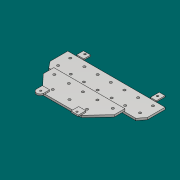
# Autodesk Inventor part: plastic_mount
Saved by Autodesk Inventor 2018 (Build 220112000, 112)
## iProperties
Created: 2021-07-30
Part Number: plastic_mount
Material: アルミニウム 6061
Document SubType Name: Modeling
Designer: gisen
Density: 2.7 g/cm^3
Appearance: アルミニウム - フラット
Author: gisen
Autodesk Inventor part; units mm, degrees
ref_plane "YZ Plane" through (0, 0, 0) normal (1, 0, 0) x (0, 1, 0)
ref_plane "XZ Plane" through (0, 0, 0) normal (0, 1, 0) x (-1, 0, 0)
ref_plane "XY Plane" through (0, 0, 0) normal (0, 0, 1) x (1, 0, 0)
sketch "スケッチ1" plane through (0, 0, 0) normal (0, 0, 1) x (1, 0, 0)
  line L0 (-67.1, 0) -> (-67.1, -24.4741)
  line L1 (-67.1, -24.4741) -> (-60, -33.4)
  line L2 (-60, -33.4) -> (60, -33.4)
  line L3 (60, -33.4) -> (67.1, -24.4741)
  line L4 (67.1, -24.4741) -> (67.1, 0)
  line L5 (67.1, 0) -> (-67.1, 0)
  line L6 (0, 0) -> (0, -33.4) construction
  circle A0 centre (0, -7.8) radius 1.65
  circle A1 centre (0, -26) radius 1.65
  circle A2 centre (18.5, -7.5) radius 1.65
  circle A3 centre (37, -7.2) radius 1.65
  circle A4 centre (19.1, -25.8) radius 1.65
  circle A5 centre (37.5, -25.5) radius 1.65
  circle A6 centre (57, -6.7) radius 1.65
  circle A7 centre (56.5, -24) radius 1.65
  circle A8 centre (-18.5, -7.5) radius 1.65
  circle A9 centre (-37, -7.2) radius 1.65
  circle A10 centre (-19.1, -25.8) radius 1.65
  circle A11 centre (-37.5, -25.5) radius 1.65
  circle A12 centre (-57, -6.7) radius 1.65
  circle A13 centre (-56.5, -24) radius 1.65
  dimension "d0" = 134.2
  dimension "d1" = 33.4
  dimension "d2" = 141.5
  dimension "d4" = 120
  dimension "d5" = 24.4741
  dimension "d6" = 6.7
  dimension "d7" = 10.1
  dimension "d8" = 7.2
  dimension "d9" = 30.1
  dimension "d10" = 48.6
  dimension "d11" = 7.5
  dimension "d12" = 7.8
  dimension "d13" = 10.6
  dimension "d14" = 24
  dimension "d15" = 29.6
  dimension "d16" = 25.5
  dimension "d17" = 25.8
  dimension "d18" = 48
  dimension "d19" = 26
  dimension "d20" = 3.3
  dimension "d21" = 37
  dimension "d22" = 74
  dimension "d23" = 114
  constraints: 14 centre point, 14 end point, 9 coincident, 7 equal radius, 6 symmetric about line, 2 equal length, 2 midpoint, 2 vertical alignment, 1 horizontal, 1 parallel, 1 perpendicular, 1 vertical, 6 other
  measures "d0" distance of L4.end L0.start
  measures "d1" distance between parallel lines of L2 L5
  measures "d2" angle of L3 L4
  measures "d4" distance of L1.end L2.end
  measures "d5" distance of L3.end L4.end
  measures "d6" distance from line of point (57, -6.7) L5
  measures "d7" distance from line of L4 point (57, -6.7)
  measures "d8" distance from line of point (37, -7.2) L5
  measures "d9" distance from line of point (37, -7.2) L4
  measures "d10" distance from line of L4 point (18.5, -7.5)
  measures "d11" distance from line of point (18.5, -7.5) L5
  measures "d12" distance from line of point (0, -7.8) L5
  measures "d13" distance from line of L4 point (56.5, -24)
  measures "d14" distance from line of point (56.5, -24) L5
  measures "d15" distance from line of L4 point (37.5, -25.5)
  measures "d16" distance from line of point (37.5, -25.5) L5
  measures "d17" distance from line of point (19.1, -25.8) L5
  measures "d18" distance from line of point (19.1, -25.8) L4
  measures "d19" distance from line of point (0, -26) L5
  measures "d20" diameter of A0
  measures "d21" distance of point (18.5, -7.5) A8.centre
  measures "d22" distance of A3.centre A9.centre
  measures "d23" distance of A6.centre A12.centre
extrude "押し出し1" add sketch "スケッチ1" along normal blind 2.8
ref_plane "作業平面1" through (0, 0, 4.5) normal (0, 0, -1) x (-1, 0, 0)
sketch "スケッチ2" plane through (0, 0, 4.5) normal (0, 0, -1) x (-1, 0, 0)
  line L0 (-67.1, 0) -> (67.1, 0) construction
  line L1 (54.9, 0) -> (45, 0)
  line L2 (45, 0) -> (45, 9.35)
  line L3 (45, 9.35) -> (54.9, 9.35)
  line L4 (54.9, 9.35) -> (54.9, 0)
  line L5 (-46.8, 0) -> (-55, 0)
  line L6 (-55, 0) -> (-55, 12.15)
  line L7 (-55, 12.15) -> (-46.8, 12.15)
  line L8 (-46.8, 12.15) -> (-46.8, 0)
  line L9 (67.1, 0) -> (67.1, -24.4741) projected
  line L10 (-67.1, -24.4741) -> (-67.1, 0) projected
  circle A0 centre (49.95, 6.45) radius 1.4
  line L11 (49.95, 6.45) -> (49.95, 7.85) construction
  line L12 (49.95, 7.85) -> (49.95, 9.35) construction
  arc A1 (-48.8, 6.45) -> (-50.2, 7.85) centre (-50.2, 6.45) ccw
  line L13 (-50.2, 6.45) -> (-50.2, 7.85) construction
  line L14 (-50.2, 6.45) -> (-48.8, 6.45) construction
  arc A2 (-50.2, 7.85) -> (-48.8, 6.45) centre (-50.2, 6.45) ccw
  line L15 (-50.2, 7.85) -> (-50.2, 12.15) construction
  line L16 (-48.8, 6.45) -> (-46.8, 6.45) construction
  point P0 (0, 0)
  dimension "d34" = 2.8
  dimension "d27" = 12.2
  dimension "d28" = 9.9
  dimension "d29" = 91.8
  dimension "d30" = 8.2
  dimension "d31" = 12.1
  dimension "d32" = 12.15
  dimension "d33" = 9.35
  dimension "d35" = 1.5
  dimension "d36" = 6.45
  dimension "d37" = 4.3
  dimension "d38" = 2
  dimension "d39" = 100.15
  constraints: 28 end point, 8 perpendicular, 4 parallel, 4 point on circle, 4 point on line, 2 centre point, 2 horizontal, 2 vertical, 1 midpoint, 1 vertical alignment, 3 other
  measures "d27" distance between parallel lines of L9 L4
  measures "d28" distance between parallel lines of L2 L4
  measures "d29" distance between parallel lines of L8 L2
  measures "d30" distance of L6.end L7.end
  measures "d31" distance between parallel lines of L10 L6
  measures "d32" distance between parallel lines of L0 L7
  measures "d33" distance between parallel lines of L0 L3
  measures "d35" distance of L11.end L12.end
  measures "d36" distance from line of L0 L11.start
  measures "d37" distance of L13.end L15.end
  measures "d38" distance of L14.end L16.end
  measures "d39" distance of L13.start L11.start
extrude "押し出し2" add sketch "スケッチ2" along normal blind 1.6
ref_plane "作業平面2" through (0, 0, 10.8) normal (0, 0, 1) x (1, 0, 0)
sketch "スケッチ3" plane through (0, 0, 10.8) normal (0, 0, 1) x (1, 0, 0)
  line L0 (-49, -37.4) -> (49, -37.4)
  line L1 (49, -37.4) -> (49, -52)
  line L2 (26.984, -75.2) -> (-26.984, -75.2)
  line L3 (-49, -52) -> (-49, -37.4)
  line L4 (-26.984, -75.2) -> (-49, -52)
  line L5 (49, -52) -> (26.984, -75.2)
  line L6 (-60, -33.4) -> (60, -33.4) construction
  circle A0 centre (0, -26) radius 1.65 construction
  circle A1 centre (0, -46.3) radius 1.65
  circle A2 centre (19.7, -46) radius 1.65
  circle A3 centre (40.3, -45.4) radius 1.65
  circle A4 centre (23.6, -64.3) radius 1.65
  circle A5 centre (0, -64.8) radius 1.65
  line L7 (0, -37.4) -> (0, -75.2) construction
  circle A6 centre (-19.7, -46) radius 1.65
  circle A7 centre (-40.3, -45.4) radius 1.65
  circle A8 centre (-23.6, -64.3) radius 1.65
  point P0 (0, 0)
  point P1 (49, -75.2)
  point P2 (-49, -75.2)
  point P3 (0, -33.4)
  dimension "d47" = 4
  dimension "d48" = 37.8
  dimension "d49" = 14.6
  dimension "d50" = 136.5
  dimension "d51" = 98
  dimension "d52" = 8
  dimension "d53" = 8.7
  dimension "d54" = 8.6
  dimension "d55" = 29.2
  dimension "d56" = 28.9
  dimension "d57" = 25.4
  dimension "d58" = 10.9
  dimension "d59" = 10.4
  dimension "d60" = 29.3
  constraints: 14 end point, 8 centre point, 5 coincident, 5 equal radius, 4 point on line, 3 midpoint, 3 symmetric about line, 3 vertical alignment, 2 equal length, 2 parallel, 1 horizontal, 1 perpendicular, 3 other
  measures "d47" distance between parallel lines of L0 L6
  measures "d48" distance between parallel lines of L2 L0
  measures "d49" distance of L0.end L1.end
  measures "d50" angle of L5 L1
  measures "d51" distance of L0.start L0.end
  measures "d52" distance from line of point (40.3, -45.4) L0
  measures "d53" distance from line of L1 point (40.3, -45.4)
  measures "d54" distance from line of point (19.7, -46) L0
  measures "d55" distance from line of L2 point (19.7, -46)
  measures "d56" distance from line of point (0, -46.3) L2
  measures "d57" distance from line of point (23.6, -64.3) L1
  measures "d58" distance from line of L2 point (23.6, -64.3)
  measures "d59" distance from line of L2 point (0, -64.8)
  measures "d60" distance from line of L1 A2.centre
extrude "押し出し3" add sketch "スケッチ3" against normal blind 2.8
ref_plane "作業平面3" through (0, 0, 16.2) normal (0, 0, 1) x (1, 0, 0)
sketch "スケッチ4" plane through (0, 0, 16.2) normal (0, 0, 1) x (1, 0, 0)
  line L0 (-30, -80.2) -> (-20, -80.2) construction
  line L1 (-20, -80.2) -> (-20, -72.2)
  line L2 (-20, -72.2) -> (-30, -72.2)
  line L3 (-30, -72.2) -> (-30, -80.2)
  line L4 (30, -72.2) -> (20, -72.2)
  line L5 (20, -72.2) -> (20, -82.7)
  line L6 (20, -82.7) -> (30, -82.7)
  line L7 (30, -82.7) -> (30, -72.2)
  line L8 (26.984, -75.2) -> (-26.984, -75.2) construction
  line L9 (26.984, -75.2) -> (-26.984, -75.2) construction
  arc A0 (-30, -80.2) -> (-20, -80.2) centre (-25, -80.2) ccw
  line L10 (-25, -80.2) -> (-25, -85.2) construction
  line L11 (-26.984, -75.2) -> (-49, -52) construction
  line L12 (49, -52) -> (26.984, -75.2) construction
  circle A1 centre (-25, -79.5) radius 1.25
  circle A2 centre (25, -79.5) radius 1.25
  line L13 (-25, -79.5) -> (-25, -78.25) construction
  line L14 (-25, -78.25) -> (-25, -72.2) construction
  point P0 (0, 0)
  point P1 (0, -75.2)
  point P2 (25, -72.2)
  dimension "d73" = 2.5
  dimension "d64" = 10
  dimension "d65" = 10
  dimension "d66" = 40
  dimension "d67" = 20
  dimension "d69" = 10
  dimension "d70" = 7.5
  dimension "d71" = 3
  dimension "d72" = 3
  dimension "d74" = 6.05
  dimension "d75" = 4.3
  constraints: 22 end point, 4 parallel, 3 midpoint, 3 point on circle, 3 vertical alignment, 2 centre point, 2 horizontal, 2 perpendicular, 1 collinear, 1 horizontal alignment, 1 vertical, 5 other
  measures "d64" distance of L0.start L0.end
  measures "d65" distance of L4.start L4.end
  measures "d66" distance between parallel lines of L1 L5
  measures "d67" distance from line of L1 point (0, -75.2)
  measures "d69" distance from line of L8 L10.end
  measures "d70" distance between parallel lines of L6 L8
  measures "d71" distance between parallel lines of L8 L2
  measures "d72" distance between parallel lines of L8 L4
  measures "d74" distance of L13.end L14.end
  measures "d75" distance from line of L13.start L8
extrude "押し出し4" add sketch "スケッチ4" against normal blind 2
equation "\"d67\" = 0.5 * d66"
